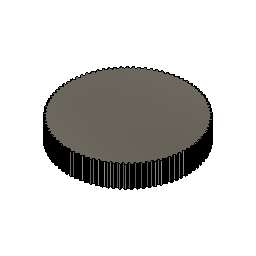
gear_87z (Autodesk Fusion 360 design; units mm, degrees)
Autodesk Fusion 360 part; units mm, degrees
sketch "Sketch1" plane through (0, 0, 0) normal (0, 0, 1) x (1, 0, 0) in component "gt2 pulley"
  circle A0 centre (0, 0) radius 27.693 construction
  circle A1 centre (0, 0) radius 26.689 construction
  line L0 (0, 0) -> (0, 27.693) construction
  line L1 (0, 0) -> (0.9998, 27.6749) construction
  line L2 (0, 0) -> (1.4045, 27.6573) construction
  circle A2 centre (0, 0) radius 27.439 construction
  arc A3 (0.3967, 27.3029) -> (0.4746, 27.0049) centre (1.3917, 27.4036) ccw
  circle A4 centre (0, 0) radius 27.289 construction
  arc A5 (0.2488, 27.4378) -> (0, 27.439) centre (0, 0) ccw
  arc A6 (0.3967, 27.3029) -> (0.2488, 27.4378) centre (0.2475, 27.2878) ccw
  arc A7 (0.4746, 27.0049) -> (0.9635, 26.6716) centre (0.9836, 27.2262) ccw
  arc A8 (0, 27.439) -> (-0.2488, 27.4378) centre (0, 0) ccw
  arc A9 (-0.2488, 27.4378) -> (-0.3967, 27.3029) centre (-0.2475, 27.2878) ccw
  arc A10 (-0.4746, 27.0049) -> (-0.3967, 27.3029) centre (-1.3917, 27.4036) ccw
  arc A11 (-0.9635, 26.6716) -> (-0.4746, 27.0049) centre (-0.9836, 27.2262) ccw
  arc A12 (0.9635, 26.6716) -> (-0.9635, 26.6716) centre (0, 0) ccw
  point P0 (1.3917, 27.4036)
  point P1 (0, 27.439)
  dimension "d18" = 55.3859
  dimension "d19" = 2.069
  dimension "d22" = 1.004
  dimension "d24" = 0.75
  dimension "d26" = 1
  dimension "d27" = 0.15
  dimension "d28" = 0.15
  dimension "d47" = 0.555
  dimension "d52" = 3.812
  constraint coincident A0.centre A1.centre
  constraint coincident A0 L0.end
  constraint vertical L0
  constraint coincident A0 L1.end
  constraint coincident A0 L2.end
  constraint concentric A1 A2
  constraint coincident A1 A7.end
  constraint coincident L1 A7.end
  constraint coincident A2 P0
  constraint coincident L2 P0
  constraint coincident P0 A3.centre
  constraint coincident A2 P1
  constraint coincident L0 P1
  constraint concentric A2 A4
  constraint coincident P1 A5.end
  constraint coincident A4 A6.centre
  constraint coincident A3.start A6.start
  constraint tangent A3 A6
  constraint tangent A3 A7
  constraint symmetric L0 A7.end A11.start
  constraint symmetric L0 A3.start A9.end
  constraint symmetric L0 A3.end A10.start
  constraint symmetric L0 A3 A10
  constraint symmetric L0 A5.start A8.end
  constraint symmetric L0 P1 A5.end
  constraint symmetric L0 A5 A8
  constraint symmetric L0 A6 A9
  constraint symmetric L0 A7 A11
  constraint coincident A1 A11.start
  constraint tangent A1 A7
  constraint coincident L1 A7.centre
  measures "d18" diameter of A0
  measures "d19" angle of L0 L1
  measures "d22" distance of A0 A1
  measures "d24" distance of A1 A2
  measures "d26" radius of A3
  measures "d27" distance of A2 A4
  measures "d28" radius of A6
  measures "d47" radius of A7
extrude "Extrude1" add sketch "Sketch1" along normal blind 10 makes body 1
pattern_circular "C-Pattern1" count 87 over 360 about axis through (0, 0, 1.75) along (0, 0, 1) of bodies 1 makes body 2 at (-2.0326, 26.6114, 6.6667) makes body 3 at (-4.5818, 26.2927, 6.6667) makes body 4 at (-5.0031, 26.2158, 6.6667) makes body 5 at (-7.5005, 25.6133, 6.6667) makes body 6 at (-8.7245, 25.2227, 3.3333) makes body 7 at (-10.5218, 24.5274, 3.3333) makes body 8 at (-13.0186, 23.2984, 6.6667) makes body 9 at (-15.1983, 21.9388, 6.6667) makes body 10 at (-16.0661, 21.3115, 6.6667) makes body 11 at (-18.1979, 19.5227, 6.6667) makes body 12 at (-19.5592, 18.1587, 6.6667) makes body 13 at (-19.8481, 17.8425, 3.3333) makes body 14 at (-21.9693, 15.1543, 6.6667) makes body 15 at (-23.0055, 13.5295, 6.6667) makes body 16 at (-23.63, 12.4066, 6.6667) makes body 17 at (-24.4636, 10.6692, 6.6667) makes body 18 at (-25.3761, 8.2677, 6.6667) makes body 19 at (-25.7446, 7.0368, 6.6667) makes body 20 at (-26.2647, 4.7399, 6.6667) makes body 21 at (-26.5601, 2.6193, 6.6667) makes body 22 at (-26.6554, 1.338, 6.6667) makes body 23 at (-26.6606, -1.231, 6.6667) makes body 24 at (-26.6374, -1.6587, 3.3333) makes body 25 at (-26.2057, -5.0557, 6.6667) makes body 26 at (-25.8274, -6.7264, 6.6667) makes body 27 at (-25.658, -7.3462, 3.3333) makes body 28 at (-25.0611, -9.1785, 3.3333) makes body 29 at (-23.6796, -12.3117, 6.6667) makes body 30 at (-23.3764, -12.8781, 6.6667) makes body 31 at (-22.0299, -15.066, 6.6667) makes body 32 at (-20.8853, -16.6164, 6.6667) makes body 33 at (-19.6319, -18.0801, 6.6667) makes body 34 at (-17.8026, -19.8838, 6.6667) makes body 35 at (-17.4812, -20.167, 3.3333) makes body 36 at (-15.2862, -21.8777, 6.6667) makes body 37 at (-14.3964, -22.4732, 3.3333) makes body 38 at (-12.7372, -23.4534, 3.3333) makes body 39 at (-11.0117, -24.3114, 3.3333) makes body 40 at (-7.8082, -25.5212, 6.6667) makes body 41 at (-5.9463, -26.0181, 6.6667) makes body 42 at (-5.528, -26.1102, 3.3333) makes body 43 at (-2.7791, -26.5439, 6.6667) makes body 44 at (-0.8565, -26.6752, 6.6667) makes body 45 at (1.0705, -26.6675, 6.6667) makes body 46 at (2.992, -26.5207, 6.6667) makes body 47 at (5.528, -26.1102, 6.6667) makes body 48 at (5.9463, -26.0181, 3.3333) makes body 49 at (7.8082, -25.5212, 3.3333) makes body 50 at (10.4233, -24.5694, 6.6667) makes body 51 at (12.7372, -23.4534, 6.6667) makes body 52 at (13.8512, -22.8132, 6.6667) makes body 53 at (15.9805, -21.3758, 6.6667) makes body 54 at (16.3214, -21.1166, 3.3333) makes body 55 at (18.8909, -18.853, 6.6667) makes body 56 at (19.7763, -17.922, 6.6667) makes body 57 at (20.4793, -17.1143, 3.3333) makes body 58 at (22.1501, -14.8887, 6.6667) makes body 59 at (22.7295, -13.9883, 3.3333) makes body 60 at (24.3334, -10.9629, 6.6667) makes body 61 at (25.0611, -9.1785, 6.6667) makes body 62 at (25.658, -7.3462, 6.6667) makes body 63 at (25.7726, -6.9335, 3.3333) makes body 64 at (26.3545, -4.2121, 6.6667) makes body 65 at (26.6374, -1.6587, 6.6667) makes body 66 at (26.6876, 0.2677, 6.6667) makes body 67 at (26.6799, 0.696, 3.3333) makes body 68 at (26.4624, 3.4703, 6.6667) makes body 69 at (26.143, 5.3708, 6.6667) makes body 70 at (25.9065, 6.4151, 3.3333) makes body 71 at (25.3761, 8.2677, 3.3333) makes body 72 at (24.3772, 10.8652, 6.6667) makes body 73 at (23.5297, 12.5958, 6.6667) makes body 74 at (22.5594, 14.2609, 6.6667) makes body 75 at (21.4716, 15.8515, 6.6667) makes body 76 at (20.2718, 17.3595, 6.6667) makes body 77 at (18.5089, 19.2282, 6.6667) makes body 78 at (17.0732, 20.5136, 6.6667) makes body 79 at (15.5484, 21.6921, 6.6667) makes body 80 at (15.1983, 21.9388, 6.6667) makes body 81 at (12.2642, 23.7042, 6.6667) makes body 82 at (10.5218, 24.5274, 6.6667) makes body 83 at (9.3291, 25.0054, 6.6667) makes body 84 at (6.8817, 25.7865, 6.6667) makes body 85 at (5.0031, 26.2158, 6.6667) makes body 86 at (4.5818, 26.2927, 3.3333) makes body 87 at (1.1775, 26.663, 6.6667)
sketch "Sketch2" plane through (0, 0, 10) normal (0, 0, 1) x (-1, 0, 0)
  arc A0 (-11.8243, -24.6129) -> (-11.7467, -24.7974) centre (-11.6825, -24.6618) ccw
  arc A1 (-11.7467, -24.7974) -> (-11.295, -25.0064) centre (0, 0) ccw
  arc A2 (-11.295, -25.0064) -> (-11.1041, -24.9461) centre (-11.2332, -24.8697) ccw
  arc A3 (-10.9083, -24.7083) -> (-11.1041, -24.9461) centre (-10.2435, -25.4552) ccw
  arc A4 (-10.3246, -24.611) -> (-10.9083, -24.7083) centre (-10.5393, -25.1228) ccw
  arc A5 (-12.0736, -23.8019) -> (-10.3246, -24.611) centre (0, 0) ccw
  arc A6 (-11.7698, -24.3097) -> (-12.0736, -23.8019) centre (-12.3247, -24.2968) ccw
  arc A7 (-11.8243, -24.6129) -> (-11.7698, -24.3097) centre (-12.7695, -24.2865) ccw
  circle A8 centre (0, 0) radius 26.689
  constraint concentric A1 A8
extrude "Extrude2" add sketch "Sketch2" against normal blind 10 contours A5 A8 bodies 1 2 3 4 5 6 7 8 9 10 11 12 13 14 15 16 17 18 19 20 21 22 23 24 25 26 27 28 29 30 31 32 33 34 35 36 37 38 39 40 41 42 43 44 45 46 47 48 49 50 51 52 53 54 55 56 57 58 59 60 61 62 63 64 65 66 67 68 69 70 71 72 73 74 75 76 77 78 79 80 81 82 83 84 85 86 87
extrude "Extrude4" [suppressed] in component "gt2 pulley"
pattern_circular "C-Pattern7" [suppressed] in component "gt2 pulley"
extrude "Extrude3" [suppressed] in component "gt2 pulley"
pattern_circular "C-Pattern6" [suppressed] in component "gt2 pulley"
extrude "Extrude2'" [suppressed] in component "gt2 pulley"
pattern_circular "C-Pattern5" [suppressed] in component "gt2 pulley"
extrude "Extrude1'" [suppressed] in component "gt2 pulley"
pattern_circular "C-Pattern4" [suppressed] in component "gt2 pulley"
pattern_circular "C-Pattern3" [suppressed] in component "gt2 pulley"
pattern_circular "C-Pattern2" [suppressed] in component "gt2 pulley"
pattern_circular "C-Pattern1'" [suppressed] in component "gt2 pulley"
copy_body "Body->Comp1" [suppressed] in component "Component"
copy_body "Body->Comp2" [suppressed] in component "Component'"
copy_body "Body->Comp3" [suppressed] in component "Component''"
copy_body "Body->Comp4" [suppressed] in component "Component'''"
copy_body "Body->Comp5" [suppressed] in component "Component''''"
copy_body "Body->Comp6" [suppressed] in component "Component'''''"
copy_body "Body->Comp7" [suppressed] in component "Component''''''"
copy_body "Body->Comp8" [suppressed] in component "Component'''''''"
copy_body "Body->Comp9" [suppressed] in component "Component''''''''"
copy_body "Body->Comp10" [suppressed] in component "Component'''''''''"
copy_body "Body->Comp11" [suppressed] in component "Component''''''''''"
copy_body "Body->Comp12" [suppressed] in component "Component'''''''''''"
copy_body "Body->Comp13" [suppressed] in component "Component''''''''''''"
copy_body "Body->Comp14" [suppressed] in component "Component'''''''''''''"
copy_body "Body->Comp15" [suppressed] in component "Component''''''''''''''"
copy_body "Body->Comp16" [suppressed] in component "Component'''''''''''''''"
copy_body "Body->Comp17" [suppressed] in component "Component''''''''''''''''"
copy_body "Body->Comp18" [suppressed] in component "Component'''''''''''''''''"
copy_body "Body->Comp19" [suppressed] in component "Component''''''''''''''''''"
copy_body "Body->Comp20" [suppressed] in component "Component'''''''''''''''''''"
component "gt2 pulley" placed x (1, 0, 0) y (0, 1, 0) z (0, 0, 1) at (0, 0, 0)
equation "NumTeeth = 87" comment "min 20"
equation "ToothPitch = 2 mm"
equation "PullyDia = NumTeeth * ToothPitch / PI"
equation "ToothAng = ( ( 360 / NumTeeth ) * 1 deg )"
equation "TransOffsetAngle = ToothAng * 0.2"
equation "Sholulder_Radius = 0.15 mm"
equation "Root_Radius = 0.555 mm"
equation "TransRadius = 1 mm"
equation "ToolHeight = 0.75 mm"
equation "PLD = 0.254 mm"
equation "d18 = PullyDia"
equation "d19 = ToothAng / 2"
equation "d22 = PLD + ToolHeight"
equation "d24 = ToolHeight"
equation "d26 = TransRadius"
equation "d27 = Sholulder_Radius"
equation "d31 = NumTeeth"
equation "d33 = NumTeeth"
equation "d35 = NumTeeth"
equation "d37 = NumTeeth"
equation "d41 = NumTeeth"
equation "d45 = NumTeeth"
equation "d47 = Root_Radius"
equation "d50 = NumTeeth"
